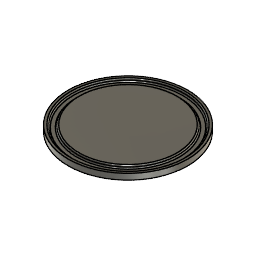
Disk (Autodesk Fusion 360 design; units mm, degrees)
Autodesk Fusion 360 part; units mm, degrees
sketch "Sketch1" plane through (0, 0, 0) normal (0, 0, 1) x (1, 0, 0)
  circle A0 centre (0, 0) radius 50
  circle A1 centre (0, 0) radius 47
  circle A2 centre (0, 0) radius 42
  dimension "d1" = 100
  dimension "d2" = -3
  dimension "d3" = -5
  constraint coincident A0.centre A1.centre
  measures "d1" diameter of A0
extrude "Extrude1" add sketch "Sketch1" along normal blind 5 contours A0 | A1 | A2
extrude "Extrude2" cut sketch "Sketch1" against normal blind 2 from surface at 5 contours A1
fillet "Fillet1" radius 1 4 edges at (-43.8194, 16.9959, 5) (-39.1577, -15.1878, 5) (-39.1577, -15.1878, 3) (-43.8194, 16.9959, 3)
